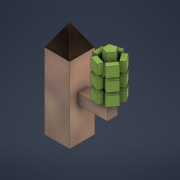
# Autodesk Inventor part: 110033226_ipt_38_小河方塊
Saved by Autodesk Inventor 2022 (Build 260153000, 153)
## iProperties
Created: 2022-06-25
Part Number: 110033226_ipt_38_小河方塊
Material: 一般
Document SubType Name: Modeling
Designer: User
Density: 1 g/cm^3
Appearance: 預設
Author: User
Autodesk Inventor part; units mm, degrees
ref_plane "YZ Plane" through (0, 0, 0) normal (1, 0, 0) x (0, 1, 0)
ref_plane "XZ Plane" through (0, 0, 0) normal (0, 1, 0) x (-1, 0, 0)
ref_plane "XY Plane" through (0, 0, 0) normal (0, 0, 1) x (1, 0, 0)
sketch "草圖1" plane through (0, 0, 0) normal (0, 1, 0) x (-1, 0, 0)
  line L0 (0, 0) -> (5, 0)
  line L1 (5, 0) -> (5, -25)
  line L2 (5, -25) -> (0, -25)
  line L3 (0, -25) -> (0, 0)
  circle A0 centre (2.5, -2.5) radius 1.7
  line L4 (5, 0) -> (0, 0)
  line L5 (0, 0) -> (0, -5)
  line L6 (0, -5) -> (5, -5)
  line L7 (5, -5) -> (5, 0)
  point P0 (5, -2.5)
  point P1 (2.5, -5)
  dimension "d0" = 5
  dimension "d1" = 25
  dimension "d2" = 3.4
  dimension "d3" = 2.5
  dimension "d4" = 2.5
  dimension "d5" = 5
  dimension "d6" = 5
  constraints: 16 end point, 4 parallel, 2 horizontal, 2 midpoint, 2 perpendicular, 1 centre point, 1 horizontal alignment, 1 vertical alignment
  measures "d0" distance of L1.end L2.end
  measures "d1" distance of L0.end L1.end
  measures "d2" diameter of A0
  measures "d3" distance from line of L3 A0.centre
  measures "d4" distance from line of L0 A0.centre
  measures "d5" distance of L6.end L5.end
  measures "d6" distance of L5.end L4.end
extrude "擠出1" add sketch "草圖1" along normal blind 15 contours L0 L1 L6 L3 | A0
sketch "草圖2" plane through (0, 0, 0) normal (1, 0, 0) x (0, 0, -1)
  line L0 (5, 15) -> (5, 0) projected
  line L1 (5, 0) -> (0, 0) projected
  line L2 (0, 0) -> (0, 15) projected
  line L3 (0, 15) -> (5, 15) projected
  line L4 (5, 15) -> (5, 0) projected
  line L5 (5, 0) -> (0, 0) projected
  line L6 (0, 0) -> (0, 15) projected
  line L7 (0, 15) -> (5, 15) projected
  line L8 (0, 0) -> (0, 15) projected
  line L9 (0, 10) -> (4, 10)
  line L10 (4, 10) -> (4, 6)
  line L11 (4, 6) -> (0, 6)
  line L12 (0, 6) -> (0, 10)
  line L13 (5, 0) -> (5, 15) projected
  line L14 (5, 10) -> (5, 6)
  line L15 (1.5, 9) -> (3.5, 9)
  line L16 (3.5, 9) -> (3.5, 7)
  line L17 (3.5, 7) -> (1.5, 7)
  line L18 (1.5, 7) -> (1.5, 9)
  point P0 (0, 0)
  point P1 (2.5, 9)
  point P2 (2.5, 15)
  point P3 (3.5, 8)
  point P4 (4, 8)
  dimension "d9" = 4
  dimension "d10" = 4
  dimension "d11" = 5
  dimension "d12" = 2
  dimension "d13" = 2
  constraints: 18 end point, 5 point on line, 4 midpoint, 4 parallel, 2 horizontal, 2 perpendicular, 1 horizontal alignment, 1 vertical alignment
  measures "d9" distance of L10.end L11.end
  measures "d10" distance of L9.end L10.end
  measures "d11" distance between parallel lines of L3 L9
  measures "d12" distance of L16.end L17.end
  measures "d13" distance of L15.end L16.end
extrude "擠出2" add sketch "草圖2" along normal blind 6 contours L15 L16 L17 L18
sketch "草圖3" plane through (0, 9, -1.5) normal (0, 1, 0) x (1, 0, 0)
  line L0 (0, -1.5) -> (-5, -1.5) projected
  line L1 (-5, -1.5) -> (-5, 3.5) projected
  line L2 (-5, 3.5) -> (0, 3.5) projected
  line L3 (0, 3.5) -> (0, 2) projected
  line L4 (0, 2) -> (0, 0) projected
  line L5 (0, 0) -> (0, -1.5) projected
  line L6 (0, 2) -> (6, 2) projected
  line L7 (6, 2) -> (6, 0) projected
  line L8 (6, 0) -> (0, 0) projected
  line L9 (6, 0) -> (5, 0)
  line L10 (5, 0) -> (5, 2)
  line L11 (5, 2) -> (6, 2)
  line L12 (6, 2) -> (6, 0)
  point P0 (0, -1.5)
  point P1 (5, 0)
  dimension "d16" = 1
  dimension "d17" = 2
  constraints: 8 end point, 2 parallel, 1 horizontal, 1 perpendicular
  measures "d16" distance of L10.end L11.end
  measures "d17" distance of L9.end L10.end
extrude "擠出3" add sketch "草圖3" along normal blind 5 contours L10 L6 L7 L8
sketch "草圖4" plane through (0, 14, -1.5) normal (0, 1, 0) x (1, 0, 0)
  line L0 (4, 0) -> (3, 0)
  line L1 (3, 0) -> (3, 2)
  line L2 (3, 2) -> (4, 2)
  line L3 (4, 2) -> (4, 0)
  line L4 (5, 2) -> (5, 0) projected
  point P0 (0, -1.5)
  point P1 (4, 1)
  point P2 (5, 1)
  dimension "d20" = 1
  dimension "d21" = 2
  dimension "d22" = 1
  constraints: 8 end point, 2 midpoint, 2 parallel, 1 horizontal, 1 horizontal alignment, 1 perpendicular
  measures "d20" distance of L1.end L2.end
  measures "d21" distance of L0.end L1.end
  measures "d22" distance between parallel lines of L4 L3
extrude "擠出4" add sketch "草圖4" along normal mid plane 2
ref_plane "工作平面1" through (0, 7, -2.5) normal (0, 0, -1) x (-1, 0, 0)
pattern_linear "矩形陣列1" count 3 spacing 2.5 along (0, 1, 0) of "擠出4" first direction both ways yes
sketch "草圖6" plane through (0, 0, 0) normal (0, -1, 0) x (1, 0, 0)
  circle A0 centre (-2.5, -2.5) radius 1.7
  line L0 (0, 0) -> (0, -5) projected
  line L1 (0, -5) -> (-5, -5) projected
  point P0 (0, 0)
  point P1 (0, -2.5)
  point P2 (-2.5, -5)
  dimension "d33" = 3.4
  constraints: 2 midpoint, 1 centre point, 1 horizontal alignment, 1 vertical alignment
  measures "d33" diameter of A0
extrude "擠出6" cut sketch "草圖6" against normal blind 1.5
sketch "草圖7" plane through (0, 15, 0) normal (0, 1, 0) x (1, 0, 0)
  line L0 (0, 0) -> (0, 5) projected
  line L1 (0, 5) -> (-5, 5) projected
  line L2 (-5, 5) -> (-5, 0) projected
  line L3 (-5, 0) -> (0, 0) projected
  point P0 (0, 0)
extrude "擠出7" add sketch "草圖7" along normal blind 10 draft -30
ref_plane "工作平面3" through (0, 7, -2.5) normal (0, 0, -1) x (-1, 0, 0)
ref_plane "工作平面4" through (5.5, 0, 0) normal (1, 0, 0) x (0, 0, -1)
pattern_circular "環形陣列2" count 5 over 360 about axis through (5.5, 7, -2.5) along (0, -1, 0) of "擠出4", "矩形陣列1"
ref_plane "工作平面5" through (4, 17.5, -1.5) normal (0, -1, 0) x (1, 0, 0)
sketch "草圖8" plane through (4, 17.5, -1.5) normal (0, -1, 0) x (1, 0, 0)
  line L0 (2.1257, 0.6907) -> (2.9348, 1.2785) projected
  line L1 (2.9348, 1.2785) -> (4.1103, -0.3396) projected
  line L2 (4.1103, -0.3396) -> (3.3013, -0.9273) projected
  line L3 (3.3013, -0.9273) -> (2.1257, 0.6907) projected
  line L4 (0.0854, 0.1176) -> (-0.2236, 1.0686) projected
  line L5 (-0.2236, 1.0686) -> (1.6785, 1.6867) projected
  line L6 (1.6785, 1.6867) -> (1.9875, 0.7356) projected
  line L7 (1.9875, 0.7356) -> (0.0854, 0.1176) projected
  line L8 (3.3013, -1.0727) -> (4.1103, -1.6604) projected
  line L9 (4.1103, -1.6604) -> (2.9348, -3.2785) projected
  line L10 (2.9348, -3.2785) -> (2.1257, -2.6907) projected
  line L11 (2.1257, -2.6907) -> (3.3013, -1.0727) projected
  line L12 (1.9875, -2.7356) -> (1.6785, -3.6867) projected
  line L13 (1.6785, -3.6867) -> (-0.2236, -3.0686) projected
  line L14 (-0.2236, -3.0686) -> (0.0854, -2.1176) projected
  line L15 (0.0854, -2.1176) -> (1.9875, -2.7356) projected
  line L16 (0, -2) -> (-1, -2) projected
  line L17 (-1, -2) -> (-1, 0) projected
  line L18 (-1, 0) -> (0, 0) projected
  line L19 (0, 0) -> (0, -2) projected
  line L20 (0.5822, -1.7328) -> (0.5822, -0.374)
  line L21 (0.5822, -0.374) -> (1.8745, 0.0459)
  line L22 (1.8745, 0.0459) -> (2.6732, -1.0534)
  line L23 (2.6732, -1.0534) -> (1.8745, -2.1527)
  line L24 (1.8745, -2.1527) -> (0.5822, -1.7328)
  line L25 (1.5174, -1.0534) -> (1.0365, 0.4266)
  line L26 (1.9875, 0.7356) -> (0.0854, 0.1176) projected
  line L27 (3.3013, -0.9273) -> (2.1257, 0.6907) projected
  point P0 (-4, 1.5)
  constraints: 12 end point, 1 midpoint, 1 parallel, 1 perpendicular, 11 other
extrude "擠出8" add sketch "草圖8" along normal mid plane 2.5 contours L20 L21 L22 L23 L24
